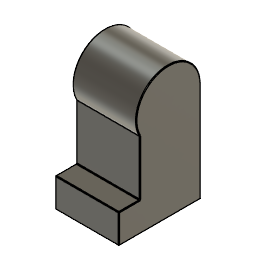
Legs (Autodesk Fusion 360 archive; units mm, degrees)
design "LeftLeg"
part number: 2026-05-19-14-25-58-594
Autodesk Fusion 360 part; units mm, degrees
sketch "LegOutline" plane through (0, 0, 0) normal (1, 0, 0) x (0, 1, 0)
  line L0 (3.5052, 0) -> (3.5052, -10.795)
  line L1 (3.5052, -10.795) -> (-5.3848, -10.795)
  line L2 (-5.3848, -10.795) -> (-5.3848, -7.62)
  line L3 (-3.0988, -1.6383) -> (-3.0988, -7.62)
  line L4 (-5.3848, -7.62) -> (-3.0988, -7.62)
  arc A0 (3.5052, 0) -> (-3.0988, -1.6383) centre (0, 0) ccw
  circle A1 centre (0, 0) radius 0.8255
  dimension "d1" = 7.0104
  dimension "d2" = 10.795
  dimension "d3" = 8.89
  dimension "d4" = 3.175
  dimension "d5" = 6.604
  dimension "d6" = 1.651
  constraint coincident A0.centre A1.centre
  constraint vertical L0
  constraint tangent L0 A0
  constraint perpendicular L0 L1
  constraint perpendicular L1 L2
  constraint vertical L3
  constraint perpendicular L3 L4
  constraint concentric A0 A1
  measures "d1" diameter of A0
  measures "d2" distance of L0.start L0.end
  measures "d3" distance of L0.end L1.end
  measures "d4" distance of L1.end L2.end
  measures "d5" distance of L0 L3
  measures "d6" diameter of A1
extrude "Extrude1" add sketch "LegOutline" against normal blind 6.9088 contours L0 L1 L2 L3 L4 A0 | A1
extrude "Extrude2" cut sketch "LegOutline" along normal blind 5.08 from surface at -6.9088 contours A1
fillet "Fillet1" radius 0.0635 2 edges at (-3.4544, -3.0988, -7.62) (-3.4544, -5.3848, -7.62) 3 faces at (-6.9088, 0.236, -6.3945) (0, 1.3039, -6.1383) (-4.6059, 0.5419, -10.795)
named bodies: "Leg"
